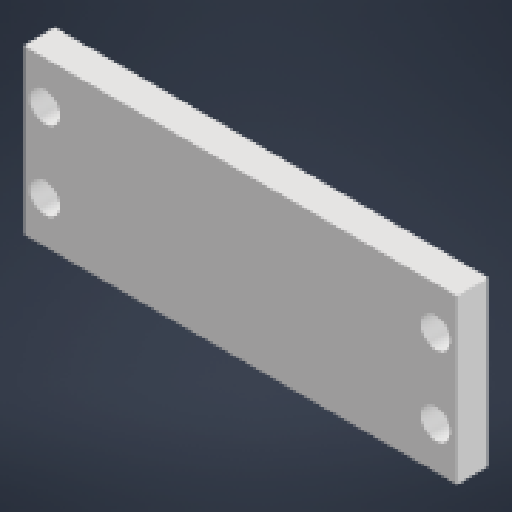
# Autodesk Inventor part: Top_Claw_Mount
Saved by Autodesk Inventor 2024.2 (Build 282272000, 272)
## iProperties
Created: 2024-06-18
Part Number: Top_Claw_Mount
Material: Generic
Document SubType Name: Modeling
Designer: warm
Density: 1 g/cm^3
Appearance: Default
Author: warm
Autodesk Inventor part; units mm, degrees
ref_plane "YZ Plane" through (0, 0, 0) normal (1, 0, 0) x (0, 1, 0)
ref_plane "XZ Plane" through (0, 0, 0) normal (0, 1, 0) x (-1, 0, 0)
ref_plane "XY Plane" through (0, 0, 0) normal (0, 0, 1) x (1, 0, 0)
sketch "Sketch1" plane through (0, 0, 0) normal (0, 0, 1) x (1, 0, 0)
  line L0 (8.55, 7) -> (8.55, 13.2) construction
  line L1 (8.55, 13.2) -> (8.1046, 13.2) construction
  arc A0 (8.1046, 13.2) -> (8.1046, 7) centre (15.75, 10.1) ccw construction
  line L2 (8.1046, 7) -> (8.55, 7) construction
  line L3 (54.5, 18.2) -> (54.5, 16.6) construction
  line L4 (54.5, 16.6) -> (53.7436, 16.6) construction
  arc A1 (53.7436, 16.6) -> (53.7436, 13.6) centre (52, 15.1) ccw construction
  line L5 (53.7436, 13.6) -> (54.5, 13.6) construction
  line L6 (54.5, 13.6) -> (54.5, 6.6) construction
  line L7 (54.5, 6.6) -> (53.7436, 6.6) construction
  arc A2 (53.7436, 6.6) -> (53.7436, 3.6) centre (52, 5.1) ccw construction
  line L8 (53.7436, 3.6) -> (54.5, 3.6) construction
  line L9 (54.5, 3.6) -> (54.5, 2) construction
  arc A3 (52.5, 0) -> (54.5, 2) centre (52.5, 2) ccw construction
  line L10 (52.5, 0) -> (46.15, 0) construction
  arc A4 (46.15, 0) -> (47.65, 1.5) centre (46.15, 1.5) ccw construction
  line L11 (47.65, 18.7) -> (47.65, 1.5) construction
  arc A5 (47.65, 18.7) -> (46.15, 20.2) centre (46.15, 18.7) ccw construction
  line L12 (8.35, 20.2) -> (46.15, 20.2)
  arc A6 (8.35, 20.2) -> (6.85, 18.7) centre (8.35, 18.7) ccw construction
  line L13 (6.85, 1.5) -> (6.85, 18.7) construction
  arc A7 (6.85, 1.5) -> (8.35, 0) centre (8.35, 1.5) ccw construction
  line L14 (8.35, 0) -> (2, 0) construction
  arc A8 (0, 2) -> (2, 0) centre (2, 2) ccw construction
  line L15 (0, 2) -> (0, 3.6) construction
  line L16 (0, 3.6) -> (0.7564, 3.6) construction
  arc A9 (0.7564, 3.6) -> (0.7564, 6.6) centre (2.5, 5.1) ccw construction
  line L17 (0.7564, 6.6) -> (0, 6.6) construction
  line L18 (0, 6.6) -> (0, 13.6) construction
  line L19 (0, 13.6) -> (0.7564, 13.6) construction
  arc A10 (0.7564, 13.6) -> (0.7564, 16.6) centre (2.5, 15.1) ccw construction
  line L20 (0.7564, 16.6) -> (0, 16.6) construction
  line L21 (0, 16.6) -> (0, 18.2) construction
  arc A11 (2, 20.2) -> (0, 18.2) centre (2, 18.2) ccw construction
  line L22 (2, 20.2) -> (8.35, 20.2)
  arc A12 (54.5, 18.2) -> (52.5, 20.2) centre (52.5, 18.2) ccw construction
  line L23 (46.15, 20.2) -> (52.5, 20.2)
  line L24 (46.15, 0) -> (8.35, 0) construction
  line L25 (54.5, 0) -> (0, 0)
  line L26 (0, 0) -> (0, 20.2) construction
  line L27 (0, 20.2) -> (54.5, 20.2) construction
  line L28 (54.5, 20.2) -> (54.5, 0) construction
  line L29 (54.75, 20.45) -> (-0.25, 20.45)
  line L30 (-0.25, 20.45) -> (-0.25, -0.25)
  line L31 (-0.25, -0.25) -> (54.75, -0.25)
  line L32 (54.75, -0.25) -> (54.75, 20.45)
  line L33 (6.6, -0.25) -> (6.6, 20.45)
  line L34 (47.9, -0.25) -> (47.9, 20.45)
  circle A13 centre (2.5, 5.1) radius 1.9
  circle A14 centre (2.5, 15.1) radius 1.9
  circle A15 centre (52, 5.1) radius 1.9
  circle A16 centre (52, 15.1) radius 1.9
  point P0 (0, 0)
  point P1 (6.6, 20.2)
  point P2 (47.9, 20.2)
  point P3 (47.9, 0)
  point P4 (6.6, 0)
  dimension "d0" = 0
  dimension "d1" = 0
  dimension "d2" = 0.25
  dimension "d3" = 0
  dimension "d4" = 0
  dimension "d5" = 0.25
  dimension "d6" = 0.25
  dimension "d7" = 3.8
  dimension "d8" = 3.8
  dimension "d9" = 3.8
  dimension "d10" = 3.8
  constraints: 70 end point, 26 point on circle, 17 centre point, 17 horizontal, 9 vertical, 6 parallel, 4 coincident, 4 point on line, 2 perpendicular, 65 other
  measures "d0" distance between parallel lines of L18 L26
  measures "d1" distance between parallel lines of L27 L22
  measures "d2" distance between parallel lines of L27 L29
  measures "d3" distance between parallel lines of L24 L25
  measures "d4" distance between parallel lines of L6 L28
  measures "d5" distance between parallel lines of L13 L33
  measures "d6" distance between parallel lines of L11 L34
  measures "d7" diameter of A13
  measures "d8" diameter of A14
  measures "d9" diameter of A15
  measures "d10" diameter of A16
extrude "Extrusion1" add sketch "Sketch1" along normal blind 7 contours L22 L33 L29 L34 L23 L12 | L33 L31 L30 L29 | L34 L29 L32 L31 | L25 L34 L31 L33
ref_plane "Work Plane1" through (65.885, 15.7373, 10.7) normal (0, 0, -1) x (0.0023, 1, 0)
sketch "Sketch3" plane through (0, 0, 0) normal (0, 0, -1) x (-1, 0, 0)
  circle A0 centre (-51.2633, 10.1) radius 7.905 construction
  line L0 (10.9433, -15.3) -> (-77.9567, -15.3) construction
  line L1 (10.9433, 35.5) -> (10.9433, -15.3) construction
  line L2 (-77.9567, 35.5) -> (10.9433, 35.5) construction
  line L3 (-77.9567, -15.3) -> (-77.9567, 35.5) construction
  circle A1 centre (-15.75, 10.1) radius 7.905 construction
  line L4 (10.9433, -15.3) -> (-77.9567, -15.3)
  line L5 (-77.9567, -15.3) -> (-77.9567, 20.45)
  line L6 (-77.9567, 20.45) -> (10.9433, 20.45)
  line L7 (10.9433, 20.45) -> (10.9433, -15.3)
  line L8 (-54.75, 20.45) -> (0.25, 20.45) projected
  circle A2 centre (-52, 5.1) radius 1.9 projected
  circle A3 centre (-52, 15.1) radius 1.9 projected
  circle A4 centre (-2.5, 15.1) radius 1.9 projected
  circle A5 centre (-2.5, 5.1) radius 1.9 projected
  line L9 (-6.6, 0) -> (-6.6, 20.2) projected
  line L10 (-6.6, 20.2) -> (-47.9, 20.2) projected
  line L11 (-47.9, 20.2) -> (-47.9, 0) projected
  line L12 (-47.9, 0) -> (-6.6, 0) projected
  line L13 (-54.75, 20.45) -> (0.25, 20.45) projected
  line L14 (0.25, 20.45) -> (0.25, -0.25) projected
  line L15 (0.25, -0.25) -> (-54.75, -0.25) projected
  line L16 (-54.75, -0.25) -> (-54.75, 20.45) projected
  line L17 (10.9433, 20.45) -> (-77.9567, 20.45)
  line L18 (-77.9567, 20.45) -> (-77.9567, 22.45)
  line L19 (-77.9567, 22.45) -> (10.9433, 22.45)
  line L20 (10.9433, 22.45) -> (10.9433, 20.45)
  point P0 (0, 0)
  point P1 (0.25, 20.45)
  dimension "d16" = 0
  dimension "d19" = 2
  constraints: 16 end point, 6 equal length, 2 perpendicular
  measures "d16" distance between parallel lines of L8 L6
  measures "d19" distance between parallel lines of L6 L19
extrude "Extrusion3" add sketch "Sketch3" against normal up to surface (7 mm away) contours L4 L5 L6 L16 L15 L14 L7 | L6 L18 L19 L20
sketch "Sketch4" plane through (0, 0, 7) normal (0, 0, 1) x (1, 0, 0)
  circle A0 centre (60.6, 3.5778) radius 1.9
  line L0 (-10.9433, 22.45) -> (77.9567, 22.45) construction
  line L1 (77.9567, 22.45) -> (77.9567, -15.3) construction
  line L2 (77.9567, -15.3) -> (-10.9433, -15.3) construction
  line L3 (-10.9433, -15.3) -> (-10.9433, 22.45) construction
  circle A1 centre (52, 5.1) radius 1.9 construction
  circle A2 centre (52, 15.1) radius 1.9 construction
  circle A3 centre (2.5, 15.1) radius 1.9 construction
  circle A4 centre (2.5, 5.1) radius 1.9 construction
  line L4 (6.6, 20.2) -> (6.6, 0) construction
  line L5 (6.6, 0) -> (47.9, 0) construction
  line L6 (47.9, 0) -> (47.9, 20.2) construction
  line L7 (47.9, 20.2) -> (6.6, 20.2) construction
  point P0 (0, 0)
  dimension "d20" = 3.8
  dimension "d21" = 18.8722
  dimension "d23" = 12.7
  constraints: 1 centre point
  measures "d20" diameter of A0
  measures "d21" distance from line of L0 A0.centre
  measures "d23" distance from line of L6 A0.centre
extrude "Extrusion4" cut sketch "Sketch4" against normal blind 6
body "Solid1"
